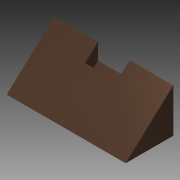
# Autodesk Inventor part: klin
Saved by Autodesk Inventor 2014 (Build 180170000, 170)
## iProperties
Created: 2013-10-18
Part Number: klin
Material: Brąz, odlew
Document SubType Name: Modeling
Designer: Wojciech
Density: 1 g/cm^3
Appearance: Brąz - satynowy
Author: Wojciech
Autodesk Inventor part; units mm, degrees
ref_plane "YZ Plane" through (0, 0, 0) normal (1, 0, 0) x (0, 1, 0)
ref_plane "XZ Plane" through (0, 0, 0) normal (0, 1, 0) x (-1, 0, 0)
ref_plane "XY Plane" through (0, 0, 0) normal (0, 0, 1) x (1, 0, 0)
sketch "Szkic1" plane through (0, 0, 0) normal (1, 0, 0) x (0, 1, 0)
  line L0 (0, 0) -> (0, 55)
  line L1 (0, 0) -> (-60, 0)
  line L2 (-60, 0) -> (0, 55)
  dimension "d0" = 55
  dimension "d1" = 60
  constraints: 6 end point, 1 perpendicular, 1 vertical
  measures "d0" distance of L0.start L0.end
  measures "d1" distance of L0.start L1.end
extrude "Wyciągnięcie proste1" add sketch "Szkic1" along normal blind 150
sketch "Szkic2" plane through (0, -60, 0) normal (0, -0.6757246, 0.7371541) x (1, 0, 0)
  line L0 (0, 81.3941) -> (150, 81.3941) projected
  line L1 (55, 81.3941) -> (95, 81.3941)
  line L2 (95, 81.3941) -> (95, 65.3941)
  line L3 (95, 65.3941) -> (55, 65.3941)
  line L4 (55, 65.3941) -> (55, 81.3941)
  point P0 (0, 44.2292)
  dimension "d4" = 40
  dimension "d5" = 16
  constraints: 8 end point, 2 parallel, 1 horizontal, 1 perpendicular, 1 point on line
  measures "d4" distance of L2.end L3.end
  measures "d5" distance of L1.end L2.end
extrude "Wyciągnięcie proste2" cut sketch "Szkic2" against normal blind 15
sketch "Szkic3" plane through (0, -60, 0) normal (0, -0.6757246, 0.7371541) x (1, 0, 0)
  line L0 (55, 65.3941) -> (95, 65.3941)
  line L1 (95, 65.3941) -> (95, 59.3941)
  line L2 (95, 59.3941) -> (55, 59.3941)
  line L3 (55, 59.3941) -> (55, 65.3941)
  point P0 (0, 44.2292)
  dimension "d8" = 40
  dimension "d9" = 6
  constraints: 8 end point, 2 parallel, 1 horizontal, 1 perpendicular
  measures "d8" distance of L1.end L2.end
  measures "d9" distance of L0.end L1.end
extrude "Wyciągnięcie proste3" cut sketch "Szkic3" against normal blind 15
sketch "Szkic4" plane through (0, -60, 0) normal (0, -0.6757246, 0.7371541) x (1, 0, 0)
  line L0 (55, 59.3941) -> (95, 59.3941)
  line L1 (95, 59.3941) -> (95, 53.3941)
  line L2 (95, 53.3941) -> (55, 53.3941)
  line L3 (55, 53.3941) -> (55, 59.3941)
  point P0 (0, 44.2292)
  dimension "d12" = 40
  dimension "d13" = 6
  constraints: 8 end point, 2 parallel, 1 horizontal, 1 perpendicular
  measures "d12" distance of L1.end L2.end
  measures "d13" distance of L0.end L1.end
extrude "Wyciągnięcie proste4" cut sketch "Szkic4" against normal blind 15
